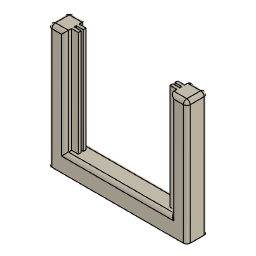
Mirror-Screen Slot Post (Autodesk Fusion 360 design; units mm, degrees)
Autodesk Fusion 360 part; units mm, degrees
imported_body "Derived Base Feature1" makes body 1
sketch "Sketch1" plane through (0, 0, 10) normal (0, 0, 1) x (-1, 0, 0)
  line L0 (-68, 29.876) -> (-68, 34.876)
  line L1 (-68, 34.876) -> (-72, 34.876)
  line L2 (-72, 34.876) -> (-72, -34.876)
  line L3 (-72, -34.876) -> (-68, -34.876)
  line L4 (-68, -34.876) -> (-68, -29.876)
  line L5 (-68, -29.876) -> (-62, -29.876)
  line L6 (-62, -29.876) -> (-62, -50.876)
  line L7 (-62, -50.876) -> (-68, -50.876)
  line L8 (-68, -50.876) -> (-68, -45.876)
  line L9 (-68, -45.876) -> (-72, -45.876)
  line L10 (-72, -45.876) -> (-72, -72)
  line L11 (-72, -72) -> (-45.876, -72)
  line L12 (-45.876, -72) -> (-45.876, -68)
  line L13 (-45.876, -68) -> (-50.876, -68)
  line L14 (-50.876, -68) -> (-50.876, -62)
  line L15 (-50.876, -62) -> (-29.876, -62)
  line L16 (-29.876, -62) -> (-29.876, -68)
  line L17 (-29.876, -68) -> (-34.876, -68)
  line L18 (-34.876, -68) -> (-34.876, -72)
  line L19 (-34.876, -72) -> (34.876, -72)
  line L20 (34.876, -72) -> (34.876, -68)
  line L21 (34.876, -68) -> (29.876, -68)
  line L22 (29.876, -68) -> (29.876, -62)
  line L23 (29.876, -62) -> (50.876, -62)
  line L24 (50.876, -62) -> (50.876, -68)
  line L25 (50.876, -68) -> (45.876, -68)
  line L26 (45.876, -68) -> (45.876, -72)
  line L27 (45.876, -72) -> (72.5, -72)
  line L28 (72.5, -72) -> (72.5, -45.126)
  line L29 (72.5, -45.126) -> (77.75, -45.126)
  line L30 (77.75, -45.126) -> (77.75, -50.126)
  line L31 (77.75, -50.126) -> (82.25, -50.126)
  line L32 (82.25, -50.126) -> (82.25, -30.626)
  line L33 (82.25, -30.626) -> (77.75, -30.626)
  line L34 (77.75, -30.626) -> (77.75, -35.626)
  line L35 (77.75, -35.626) -> (72.5, -35.626)
  line L36 (72.5, -35.626) -> (72.5, 35.626)
  line L37 (72.5, 35.626) -> (77.75, 35.626)
  line L38 (77.75, 35.626) -> (77.75, 30.626)
  line L39 (77.75, 30.626) -> (82.25, 30.626)
  line L40 (82.25, 30.626) -> (82.25, 50.126)
  line L41 (82.25, 50.126) -> (77.75, 50.126)
  line L42 (77.75, 50.126) -> (77.75, 45.126)
  line L43 (77.75, 45.126) -> (72.5, 45.126)
  line L44 (72.5, 45.126) -> (72.5, 72.5)
  line L45 (72.5, 72.5) -> (45.126, 72.5)
  line L46 (45.126, 72.5) -> (45.126, 77.75)
  line L47 (45.126, 77.75) -> (50.126, 77.75)
  line L48 (50.126, 77.75) -> (50.126, 82.25)
  line L49 (50.126, 82.25) -> (30.626, 82.25)
  line L50 (30.626, 82.25) -> (30.626, 77.75)
  line L51 (30.626, 77.75) -> (35.626, 77.75)
  line L52 (35.626, 77.75) -> (35.626, 72.5)
  line L53 (35.626, 72.5) -> (-35.626, 72.5)
  line L54 (-35.626, 72.5) -> (-35.626, 77.75)
  line L55 (-35.626, 77.75) -> (-30.626, 77.75)
  line L56 (-30.626, 77.75) -> (-30.626, 82.25)
  line L57 (-30.626, 82.25) -> (-50.126, 82.25)
  line L58 (-50.126, 82.25) -> (-50.126, 77.75)
  line L59 (-50.126, 77.75) -> (-45.126, 77.75)
  line L60 (-45.126, 77.75) -> (-45.126, 72.5)
  line L61 (-45.126, 72.5) -> (-72, 72.5)
  line L62 (-72, 72.5) -> (-72, 45.876)
  line L63 (-72, 45.876) -> (-68, 45.876)
  line L64 (-68, 45.876) -> (-68, 50.876)
  line L65 (-68, 50.876) -> (-62, 50.876)
  line L66 (-62, 50.876) -> (-62, 29.876)
  line L67 (-62, 29.876) -> (-68, 29.876)
  circle A0 centre (40.376, 40.376) radius 5.25
  circle A1 centre (-40.376, -40.376) radius 5.25
  circle A2 centre (0, -40.376) radius 5.25
  circle A3 centre (40.376, 0) radius 5.25
  circle A4 centre (0, 40.376) radius 5.25
  circle A5 centre (-40.376, 0) radius 5.25
  circle A6 centre (40.376, -40.376) radius 5.25
  circle A7 centre (0, 0) radius 5.25
  circle A8 centre (-40.376, 40.376) radius 5.25
  line L68 (-50, -7.5) -> (50, -7.5)
  line L69 (50, -7.5) -> (50, 7.5)
  line L70 (50, 7.5) -> (-50, 7.5)
  line L71 (-50, 7.5) -> (-50, -7.5)
  line L72 (-50, -7.5) -> (50, 7.5) construction
  line L73 (50, -7.5) -> (-50, 7.5) construction
  circle A9 centre (40.376, 0) radius 5.25
  circle A10 centre (-40.376, 0) radius 5.25
  dimension "d1" = 100
  dimension "d2" = 15
  constraint horizontal L68
  constraint perpendicular L68 L69
  constraint parallel L68 L70
  constraint parallel L69 L71
  constraint coincident L72 A7.centre
  constraint coincident L73 A7.centre
  constraint coincident A7.centre origin
  constraint concentric A3 A9
  constraint concentric A5 A10
  measures "d1" distance of L69.end L70.end
  measures "d2" distance of L68.end L69.end
extrude "Extrude1" add sketch "Sketch1" along normal blind 81.2 separate body contours A3 A9 | A5 A10 | A7 | L68 L69 L70 L71 makes body 2
extrude "Extrude2" cut sketch "Sketch1" along normal blind 10 contours A3 A9 | A5 A10 bodies 2
extrude "Extrude3" add 1 faces at (16.6667, -2.5, 91.2) along direction (0, 0, 1) blind 8 on bodies 2 bodies 2
sketch "Sketch2" plane through (0, 0, 99.2) normal (0, 0, 1) x (-1, 0, 0)
  line L0 (-50, 7.5) -> (-50, -7.5)
  line L1 (-50, -7.5) -> (50, -7.5)
  line L2 (50, -7.5) -> (50, 7.5)
  line L3 (50, 7.5) -> (-50, 7.5)
  line L4 (-38.1, 0.25) -> (38.1, 0.25)
  line L5 (38.1, 0.25) -> (38.1, -0.25)
  line L6 (38.1, -0.25) -> (-38.1, -0.25)
  line L7 (-38.1, -0.25) -> (-38.1, 0.25)
  line L8 (-38.1, 0.25) -> (38.1, -0.25) construction
  line L9 (38.1, 0.25) -> (-38.1, -0.25) construction
  line L10 (38.1, -0.25) -> (33.1, -0.25)
  line L11 (33.1, -0.25) -> (33.1, -2.75)
  line L12 (33.1, -2.75) -> (38.1, -2.75)
  line L13 (38.1, -2.75) -> (38.1, -0.25)
  line L14 (38.1, -2.75) -> (38.1, -7.5)
  line L15 (38.1, 0.25) -> (38.1, 7.5)
  line L16 (-38.1, 0.25) -> (-38.1, 7.5)
  line L17 (-38.1, -0.25) -> (-38.1, -7.5)
  line L18 (33.1, 0.25) -> (38.1, 0.25)
  line L19 (38.1, 0.25) -> (38.1, 2.75)
  line L20 (38.1, 2.75) -> (33.1, 2.75)
  line L21 (33.1, 2.75) -> (33.1, 0.25)
  line L22 (-38.1, 0.25) -> (-33.1, 0.25)
  line L23 (-33.1, 0.25) -> (-33.1, 2.75)
  line L24 (-33.1, 2.75) -> (-38.1, 2.75)
  line L25 (-38.1, 2.75) -> (-38.1, 0.25)
  line L26 (-38.1, -0.25) -> (-33.1, -0.25)
  line L27 (-33.1, -0.25) -> (-33.1, -2.75)
  line L28 (-33.1, -2.75) -> (-38.1, -2.75)
  line L29 (-38.1, -2.75) -> (-38.1, -0.25)
  dimension "d9" = 76.2
  dimension "d10" = 0.5
  dimension "d11" = 5
  dimension "d12" = 2.5
  dimension "d13" = 2.5
  dimension "d14" = 5
  dimension "d15" = 2.5
  dimension "d16" = 5
  dimension "d17" = 2.5
  constraint horizontal L4
  constraint perpendicular L4 L5
  constraint parallel L4 L6
  constraint parallel L5 L7
  constraint coincident L8 origin
  constraint coincident L9 origin
  constraint horizontal L10
  constraint vertical L11
  constraint horizontal L12
  constraint vertical L13
  constraint coincident L1 L14.end
  constraint perpendicular L1 L14
  constraint coincident L3 L15.end
  constraint perpendicular L3 L15
  constraint coincident L3 L16.end
  constraint perpendicular L3 L16
  constraint coincident L1 L17.end
  constraint perpendicular L1 L17
  constraint horizontal L18
  constraint vertical L19
  constraint horizontal L20
  constraint vertical L21
  constraint coincident L4 L18.start
  constraint horizontal L22
  constraint vertical L23
  constraint horizontal L24
  constraint vertical L25
  constraint horizontal L26
  constraint vertical L27
  constraint horizontal L28
  constraint vertical L29
  measures "d9" distance of L5.end L6.end
  measures "d10" distance of L4.end L5.end
  measures "d11" distance of L5.end L10.end
  measures "d12" distance of L5.end L12.end
  measures "d13" distance of L18.start L20.end
  measures "d14" distance of L4.start L22.end
  measures "d15" distance of L4.start L24.end
  measures "d16" distance of L6.end L26.end
  measures "d17" distance of L6.end L28.end
extrude "Extrude4" cut sketch "Sketch2" against normal blind 76.2 contours L3 L4 L15 L16 L20 L21 L23 L24 | L1 L6 L11 L12 L14 L17 L27 L28 | L4 L5 L6 L7 L10 L18 L22 L26 bodies 2
fillet "Fillet1" radius 2.5 16 edges at (-38.1, -7.5, 61.1) (0, -7.5, 23) (38.1, -7.5, 61.1) (50, -7.5, 54.6) (50, 7.5, 54.6) (-50, -7.5, 54.6) (-50, 7.5, 54.6) (0, 7.5, 23) (38.1, 7.5, 61.1) (-38.1, 7.5, 61.1) (-44.05, 7.5, 99.2) (-50, 0, 99.2) (-44.05, -7.5, 99.2) (44.05, -7.5, 99.2) (50, 0, 99.2) (44.05, 7.5, 99.2) on bodies 2
extrude "Extrude5" cut 1 faces at (-36.4333, 0.25, 48.4) along direction (0, 1, 0) blind 0.375 on bodies 2 bodies 2
extrude "Extrude6" cut 1 faces at (-34.7667, -0.25, 48.4) along direction (0, -1, 0) blind 0.375 on bodies 2 bodies 2
extrude "Extrude7" cut 1 faces at (34.7667, 0.25, 48.4) along direction (0, 1, 0) blind 0.375 on bodies 2 bodies 2
extrude "Extrude8" cut 1 faces at (36.4333, -0.25, 48.4) along direction (0, -1, 0) blind 0.375 on bodies 2 bodies 2
extrude "Extrude9" cut 1 faces at (-36.4333, 0.625, 48.4) along direction (0, 1, 0) blind 0.125 on bodies 2 bodies 2
extrude "Extrude10" cut 1 faces at (-34.7667, -0.625, 48.4) along direction (0, -1, 0) blind 0.125 on bodies 2 bodies 2
extrude "Extrude11" cut 1 faces at (36.4333, -0.625, 48.4) along direction (0, -1, 0) blind 0.125 on bodies 2 bodies 2
extrude "Extrude12" cut 1 faces at (34.7667, 0.625, 48.4) along direction (0, 1, 0) blind 0.125 on bodies 2 bodies 2
hidden bodies 1
named bodies: "Optical Breadboard", "Mirror Slot Post"
